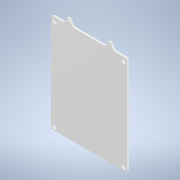
# Autodesk Inventor part: back plate
Saved by Autodesk Inventor 2022 (Build 260153000, 153)
## iProperties
Created: 2021-05-28
Part Number: back plate
Material: ABS Plastic
Document SubType Name: Modeling
Designer: benka
Density: 1.06 g/cm^3
Appearance: Smooth - White
Author: benka
Autodesk Inventor part; units mm, degrees
ref_plane "YZ Plane" through (0, 0, 0) normal (1, 0, 0) x (0, 1, 0)
ref_plane "XZ Plane" through (0, 0, 0) normal (0, 1, 0) x (-1, 0, 0)
ref_plane "XY Plane" through (0, 0, 0) normal (0, 0, 1) x (1, 0, 0)
sketch "Sketch1" plane through (0, 0, 0) normal (0, 0, 1) x (1, 0, 0)
  ellipse E0 centre (-53.6, 142.4744) end of major axis (-55.5943, 142.4744) minor radius 1.993
  ellipse E1 centre (53.6, 142.4744) end of major axis (51.6057, 142.4744) minor radius 1.993
  line L0 (-57.5, 147.4744) -> (-50, 147.4744)
  line L1 (50, 147.4744) -> (57.5, 147.4744)
  line L2 (99, 127.7477) -> (99, -119.2334)
  line L3 (-99, 127.7477) -> (-99, -119.2334)
  line L4 (-94, -124.2334) -> (94, -124.2334)
  line L5 (94, 132.7477) -> (72, 132.7477)
  line L6 (57.5, 147.2477) -> (57.5, 147.4744)
  line L7 (50, 147.4744) -> (50, 147.2477)
  line L8 (35.5, 132.7477) -> (-35.5, 132.7477)
  line L9 (-50, 147.2477) -> (-50, 147.4744)
  line L10 (-57.5, 147.4744) -> (-57.5, 147.2477)
  line L11 (-72, 132.7477) -> (-94, 132.7477)
  arc A0 (57.5, 147.2477) -> (72, 132.7477) centre (72, 147.2477) ccw
  arc A1 (35.5, 132.7477) -> (50, 147.2477) centre (35.5, 147.2477) ccw
  arc A2 (-50, 147.2477) -> (-35.5, 132.7477) centre (-35.5, 147.2477) ccw
  arc A3 (-72, 132.7477) -> (-57.5, 147.2477) centre (-72, 147.2477) ccw
  arc A4 (99, 127.7477) -> (94, 132.7477) centre (94, 127.7477) ccw
  arc A5 (-94, 132.7477) -> (-99, 127.7477) centre (-94, 127.7477) ccw
  arc A6 (94, -124.2334) -> (99, -119.2334) centre (94, -119.2334) ccw
  arc A7 (-99, -119.2334) -> (-94, -124.2334) centre (-94, -119.2334) ccw
  circle A8 centre (90.0016, 122.2919) radius 5
  circle A9 centre (-89.9984, 122.2919) radius 5
  circle A10 centre (90.0016, -116.3073) radius 5
  circle A11 centre (-89.9984, -116.3073) radius 5
  point P0 (57.5, 132.7477)
  point P1 (-57.5, 132.7477)
  point P2 (-99, 132.7477)
  dimension "d3" = 7.5
  dimension "d4" = 7.5
  dimension "d18" = 5
  dimension "d28" = 14.7267
  dimension "d29" = 14.5
  dimension "d31" = 5
  constraints: 24 end point, 16 point on circle, 16 tangent, 12 centre point, 7 point on line, 6 equal radius, 3 perpendicular, 2 collinear, 1 horizontal, 1 parallel, 1 vertical, 12 other
  measures "d3" distance of L0.start L0.end
  measures "d4" distance of L1.end L1.start
  measures "d18" distance from line of L1 point (53.6, 142.474)
  measures "d28" distance of point (57.5, 132.748) L1.end
  measures "d29" radius of A0
  measures "d31" radius of A4
extrude "Extrusion1" add sketch "Sketch1" along normal blind 5
body "Solid1"
